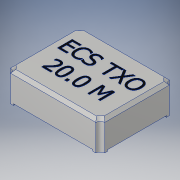
# Autodesk Inventor part: Crystal_TXO-3225
Saved by Autodesk Inventor 2018 (Build 220112000, 112)
## iProperties
Created: 2016-08-15
Part Number: Crystal_TXO-3225
Material: Aluminum 6061
Document SubType Name: Modeling
Designer: Bradley
Density: 2.7 g/cm^3
Appearance: Aluminum - Flat
Author: Bradley
Autodesk Inventor part; units mm, degrees
ref_plane "YZ Plane" through (0, 0, 0) normal (1, 0, 0) x (0, 1, 0)
ref_plane "XZ Plane" through (0, 0, 0) normal (0, 1, 0) x (-1, 0, 0)
ref_plane "XY Plane" through (0, 0, 0) normal (0, 0, 1) x (1, 0, 0)
sketch "Sketch1" plane through (0, 0, 0) normal (0, 1, 0) x (-1, 0, 0)
  line L0 (-1.6, 1.25) -> (1.6, 1.25)
  line L1 (1.6, 1.25) -> (1.6, -1.25)
  line L2 (1.6, -1.25) -> (-1.6, -1.25)
  line L3 (-1.6, -1.25) -> (-1.6, 1.25)
  line L4 (-1.6, 1.25) -> (1.6, -1.25) construction
  line L5 (1.6, 1.25) -> (-1.6, -1.25) construction
  arc A0 (1.6, -1.1) -> (1.45, -1.25) centre (1.6, -1.25) ccw
  arc A1 (-1.45, -1.25) -> (-1.6, -1.1) centre (-1.6, -1.25) ccw
  arc A2 (-1.6, 1.1) -> (-1.45, 1.25) centre (-1.6, 1.25) ccw
  arc A3 (1.45, 1.25) -> (1.6, 1.1) centre (1.6, 1.25) ccw
  point P0 (0, 0)
  dimension "d0" = 3.2
  dimension "d1" = 2.5
  dimension "d4" = 0.15
  constraints: 12 end point, 8 point on circle, 8 point on line, 4 centre point, 4 coincident, 3 equal radius, 2 midpoint, 2 parallel, 1 horizontal, 1 perpendicular
  measures "d0" distance of L1.end L2.end
  measures "d1" distance of L0.end L1.end
  measures "d4" radius of A0
extrude "Extrusion1" add sketch "Sketch1" along normal mid plane 0.95 contours L0 A3 L1 A0 L2 A1 L3 A2
chamfer "Chamfer1" distance 0.1 angle 45 8 edges at (0, 0.475, 1.25) (-1.4939, 0.475, 1.1439) (-1.6, 0.475, 0) (-1.4939, 0.475, -1.1439) (0, 0.475, -1.25) (1.4939, 0.475, -1.1439) (1.6, 0.475, 0) (1.4939, 0.475, 1.1439)
sketch "Sketch3" plane through (0, 0.475, 0) normal (0, 1, 0) x (1, 0, 0)
  line L0 (-1.3709, 1.15) -> (1.3709, 1.15) projected
  arc A0 (-1.5, 1.0209) -> (-1.3709, 1.15) centre (-1.6, 1.25) ccw projected
  line L1 (-1.5, -1.0209) -> (-1.5, 1.0209) projected
  arc A1 (-1.3709, -1.15) -> (-1.5, -1.0209) centre (-1.6, -1.25) ccw projected
  line L2 (1.3709, -1.15) -> (-1.3709, -1.15) projected
  arc A2 (1.5, -1.0209) -> (1.3709, -1.15) centre (1.6, -1.25) ccw projected
  line L3 (1.5, 1.0209) -> (1.5, -1.0209) projected
  arc A3 (1.3709, 1.15) -> (1.5, 1.0209) centre (1.6, 1.25) ccw projected
  line L4 (1.5, 1.0209) -> (1.5, -1.0209) construction
  line L5 (1.5, 0.1868) -> (-1.5, 0.1868) construction
  line L6 (-1.2911, 0.1868) -> (-1.2911, 0.6868)
  line L7 (-1.2911, 0.6868) -> (-0.9783, 0.6868)
  line L8 (-0.9783, 0.6868) -> (-0.9783, 0.6276)
  line L9 (-0.9783, 0.6276) -> (-1.2247, 0.6276)
  line L10 (-1.2247, 0.6276) -> (-1.2247, 0.4906)
  line L11 (-1.2247, 0.4906) -> (-0.9949, 0.4906)
  line L12 (-0.9949, 0.4906) -> (-0.9949, 0.4315)
  line L13 (-0.9949, 0.4315) -> (-1.2247, 0.4315)
  line L14 (-1.2247, 0.4315) -> (-1.2247, 0.2459)
  line L15 (-1.2247, 0.2459) -> (-0.9783, 0.2459)
  line L16 (-0.9783, 0.2459) -> (-0.9783, 0.1868)
  line L17 (-0.9783, 0.1868) -> (-1.2911, 0.1868)
  spline S0 degree 2 poles (-0.7101, 0.1778) (-0.7587, 0.1778) (-0.841, 0.2107) (-0.8709, 0.2435) knots 0 0 0 1 2 2 2
  spline S1 degree 2 poles (-0.8709, 0.2435) (-0.9009, 0.2759) (-0.9338, 0.3731) (-0.9338, 0.4364) knots 0 0 0 1 2 2 2
  spline S2 degree 2 poles (-0.9338, 0.4364) (-0.9338, 0.4992) (-0.9017, 0.5923) (-0.8714, 0.6268) knots 0 0 0 1 2 2 2
  spline S3 degree 2 poles (-0.8714, 0.6268) (-0.8414, 0.6604) (-0.7595, 0.6957) (-0.7089, 0.6957) knots 0 0 0 1 2 2 2
  spline S4 degree 2 poles (-0.7089, 0.6957) (-0.6838, 0.6957) (-0.6396, 0.6884) (-0.6209, 0.6827) knots 0 0 0 1 2 2 2
  spline S5 degree 2 poles (-0.6209, 0.6827) (-0.6047, 0.6774) (-0.5711, 0.6624) (-0.5545, 0.6535) knots 0 0 0 1 2 2 2
  line L18 (-0.5545, 0.6535) -> (-0.5545, 0.5733)
  line L19 (-0.5545, 0.5733) -> (-0.5598, 0.5733)
  spline S6 degree 2 poles (-0.5598, 0.5733) (-0.5687, 0.5814) (-0.5962, 0.6041) (-0.6161, 0.615) knots 0 0 0 1 2 2 2
  spline S7 degree 2 poles (-0.6161, 0.615) (-0.6351, 0.6256) (-0.6801, 0.6389) (-0.7093, 0.6389) knots 0 0 0 1 2 2 2
  spline S8 degree 2 poles (-0.7093, 0.6389) (-0.7413, 0.6389) (-0.7984, 0.6126) (-0.8199, 0.5875) knots 0 0 0 1 2 2 2
  spline S9 degree 2 poles (-0.8199, 0.5875) (-0.841, 0.562) (-0.8645, 0.4846) (-0.8645, 0.4364) knots 0 0 0 1 2 2 2
  spline S10 degree 2 poles (-0.8645, 0.4364) (-0.8645, 0.3849) (-0.8397, 0.3107) (-0.8183, 0.2852) knots 0 0 0 1 2 2 2
  spline S11 degree 2 poles (-0.8183, 0.2852) (-0.7972, 0.2605) (-0.7409, 0.2354) (-0.7093, 0.2354) knots 0 0 0 1 2 2 2
  spline S12 degree 2 poles (-0.7093, 0.2354) (-0.6805, 0.2354) (-0.6315, 0.2496) (-0.6124, 0.2601) knots 0 0 0 1 2 2 2
  spline S13 degree 2 poles (-0.6124, 0.2601) (-0.5942, 0.2706) (-0.5671, 0.2925) (-0.5594, 0.3002) knots 0 0 0 1 2 2 2
  line L20 (-0.5594, 0.3002) -> (-0.5545, 0.3002)
  line L21 (-0.5545, 0.3002) -> (-0.5545, 0.2208)
  spline S14 degree 2 poles (-0.5545, 0.2208) (-0.5711, 0.2131) (-0.6003, 0.1989) (-0.6209, 0.1924) knots 0 0 0 1 2 2 2
  spline S15 degree 2 poles (-0.6209, 0.1924) (-0.6428, 0.1851) (-0.6801, 0.1778) (-0.7101, 0.1778) knots 0 0 0 1 2 2 2
  spline S16 degree 2 poles (-0.3531, 0.1778) (-0.4074, 0.1778) (-0.4836, 0.2005) (-0.5172, 0.2167) knots 0 0 0 1 2 2 2
  line L22 (-0.5172, 0.2167) -> (-0.5172, 0.3002)
  line L23 (-0.5172, 0.3002) -> (-0.5124, 0.3002)
  spline S17 degree 2 poles (-0.5124, 0.3002) (-0.4795, 0.2694) (-0.3965, 0.2354) (-0.358, 0.2354) knots 0 0 0 1 2 2 2
  spline S18 degree 2 poles (-0.358, 0.2354) (-0.3029, 0.2354) (-0.2466, 0.2812) (-0.2466, 0.3188) knots 0 0 0 1 2 2 2
  spline S19 degree 2 poles (-0.2466, 0.3188) (-0.2466, 0.3488) (-0.2761, 0.3861) (-0.3081, 0.3954) knots 0 0 0 1 2 2 2
  spline S20 degree 2 poles (-0.3081, 0.3954) (-0.3312, 0.4019) (-0.3697, 0.4108) (-0.3985, 0.4181) knots 0 0 0 1 2 2 2
  spline S21 degree 2 poles (-0.3985, 0.4181) (-0.4244, 0.425) (-0.4654, 0.4457) (-0.4812, 0.4623) knots 0 0 0 1 2 2 2
  spline S22 degree 2 poles (-0.4812, 0.4623) (-0.4966, 0.4789) (-0.5136, 0.5235) (-0.5136, 0.5526) knots 0 0 0 1 2 2 2
  spline S23 degree 2 poles (-0.5136, 0.5526) (-0.5136, 0.6134) (-0.4188, 0.6957) (-0.3454, 0.6957) knots 0 0 0 1 2 2 2
  spline S24 degree 2 poles (-0.3454, 0.6957) (-0.3033, 0.6957) (-0.2287, 0.6791) (-0.1967, 0.6633) knots 0 0 0 1 2 2 2
  line L24 (-0.1967, 0.6633) -> (-0.1967, 0.5838)
  line L25 (-0.1967, 0.5838) -> (-0.2016, 0.5838)
  spline S25 degree 2 poles (-0.2016, 0.5838) (-0.2255, 0.6057) (-0.3, 0.6381) (-0.341, 0.6381) knots 0 0 0 1 2 2 2
  spline S26 degree 2 poles (-0.341, 0.6381) (-0.3872, 0.6381) (-0.4443, 0.5948) (-0.4443, 0.5595) knots 0 0 0 1 2 2 2
  spline S27 degree 2 poles (-0.4443, 0.5595) (-0.4443, 0.5279) (-0.4107, 0.4902) (-0.3791, 0.4817) knots 0 0 0 1 2 2 2
  spline S28 degree 2 poles (-0.3791, 0.4817) (-0.358, 0.4761) (-0.2968, 0.4615) (-0.2765, 0.4554) knots 0 0 0 1 2 2 2
  spline S29 degree 2 poles (-0.2765, 0.4554) (-0.2251, 0.4396) (-0.1773, 0.376) (-0.1773, 0.3294) knots 0 0 0 1 2 2 2
  spline S30 degree 2 poles (-0.1773, 0.3294) (-0.1773, 0.2998) (-0.2012, 0.2431) (-0.2226, 0.2232) knots 0 0 0 1 2 2 2
  spline S31 degree 2 poles (-0.2226, 0.2232) (-0.2466, 0.2013) (-0.3073, 0.1778) (-0.3531, 0.1778) knots 0 0 0 1 2 2 2
  line L26 (0.2218, 0.1868) -> (0.2218, 0.6276)
  line L27 (0.2218, 0.6276) -> (0.0541, 0.6276)
  line L28 (0.0541, 0.6276) -> (0.0541, 0.6868)
  line L29 (0.0541, 0.6868) -> (0.456, 0.6868)
  line L30 (0.456, 0.6868) -> (0.456, 0.6276)
  line L31 (0.456, 0.6276) -> (0.2883, 0.6276)
  line L32 (0.2883, 0.6276) -> (0.2883, 0.1868)
  line L33 (0.2883, 0.1868) -> (0.2218, 0.1868)
  line L34 (0.8527, 0.1868) -> (0.7765, 0.1868)
  line L35 (0.7765, 0.1868) -> (0.655, 0.3861)
  line L36 (0.655, 0.3861) -> (0.531, 0.1868)
  line L37 (0.531, 0.1868) -> (0.4593, 0.1868)
  line L38 (0.4593, 0.1868) -> (0.6185, 0.4372)
  line L39 (0.6185, 0.4372) -> (0.4641, 0.6868)
  line L40 (0.4641, 0.6868) -> (0.5403, 0.6868)
  line L41 (0.5403, 0.6868) -> (0.6594, 0.4911)
  line L42 (0.6594, 0.4911) -> (0.781, 0.6868)
  line L43 (0.781, 0.6868) -> (0.8527, 0.6868)
  line L44 (0.8527, 0.6868) -> (0.6963, 0.4404)
  line L45 (0.6963, 0.4404) -> (0.8527, 0.1868)
  spline S32 degree 2 poles (1.2599, 0.6296) (1.2883, 0.5964) (1.3199, 0.4992) (1.3199, 0.4368) knots 0 0 0 1 2 2 2
  spline S33 degree 2 poles (1.3199, 0.4368) (1.3199, 0.376) (1.2891, 0.2775) (1.2599, 0.2443) knots 0 0 0 1 2 2 2
  spline S34 degree 2 poles (1.2599, 0.2443) (1.2291, 0.2094) (1.1477, 0.1762) (1.0987, 0.1762) knots 0 0 0 1 2 2 2
  spline S35 degree 2 poles (1.0987, 0.1762) (1.048, 0.1762) (0.967, 0.2107) (0.9374, 0.2443) knots 0 0 0 1 2 2 2
  spline S36 degree 2 poles (0.9374, 0.2443) (0.9086, 0.2775) (0.8778, 0.3752) (0.8778, 0.4368) knots 0 0 0 1 2 2 2
  spline S37 degree 2 poles (0.8778, 0.4368) (0.8778, 0.4996) (0.909, 0.5952) (0.9378, 0.6296) knots 0 0 0 1 2 2 2
  spline S38 degree 2 poles (0.9378, 0.6296) (0.967, 0.6629) (1.0484, 0.6973) (1.0987, 0.6973) knots 0 0 0 1 2 2 2
  spline S39 degree 2 poles (1.0987, 0.6973) (1.1497, 0.6973) (1.2316, 0.6616) (1.2599, 0.6296) knots 0 0 0 1 2 2 2
  spline S40 degree 2 poles (1.2506, 0.4368) (1.2506, 0.4862) (1.2291, 0.5628) (1.2097, 0.5879) knots 0 0 0 1 2 2 2
  spline S41 degree 2 poles (1.2097, 0.5879) (1.1898, 0.6138) (1.1339, 0.6398) (1.0991, 0.6398) knots 0 0 0 1 2 2 2
  spline S42 degree 2 poles (1.0991, 0.6398) (1.063, 0.6398) (1.0087, 0.6146) (0.988, 0.5879) knots 0 0 0 1 2 2 2
  spline S43 degree 2 poles (0.988, 0.5879) (0.9682, 0.5624) (0.9471, 0.4854) (0.9471, 0.4368) knots 0 0 0 1 2 2 2
  spline S44 degree 2 poles (0.9471, 0.4368) (0.9471, 0.3383) (1.0298, 0.2338) (1.0991, 0.2338) knots 0 0 0 1 2 2 2
  spline S45 degree 2 poles (1.0991, 0.2338) (1.1684, 0.2338) (1.2506, 0.3383) (1.2506, 0.4368) knots 0 0 0 1 2 2 2
  line L46 (-0.6945, -0.6389) -> (-1.0028, -0.6389)
  line L47 (-1.0028, -0.6389) -> (-1.0028, -0.568)
  spline S46 degree 2 poles (-1.0028, -0.568) (-0.9696, -0.5368) (-0.9105, -0.4789) (-0.8821, -0.4477) knots 0 0 0 1 2 2 2
  spline S47 degree 2 poles (-0.8821, -0.4477) (-0.825, -0.3849) (-0.7832, -0.3095) (-0.7832, -0.2694) knots 0 0 0 1 2 2 2
  spline S48 degree 2 poles (-0.7832, -0.2694) (-0.7832, -0.2483) (-0.7962, -0.2167) (-0.8079, -0.2066) knots 0 0 0 1 2 2 2
  spline S49 degree 2 poles (-0.8079, -0.2066) (-0.8197, -0.1965) (-0.8505, -0.1863) (-0.8691, -0.1863) knots 0 0 0 1 2 2 2
  spline S50 degree 2 poles (-0.8691, -0.1863) (-0.887, -0.1863) (-0.9234, -0.1952) (-0.94, -0.2021) knots 0 0 0 1 2 2 2
  spline S51 degree 2 poles (-0.94, -0.2021) (-0.9542, -0.2078) (-0.9806, -0.224) (-0.9887, -0.2297) knots 0 0 0 1 2 2 2
  line L48 (-0.9887, -0.2297) -> (-0.9923, -0.2297)
  line L49 (-0.9923, -0.2297) -> (-0.9923, -0.1584)
  spline S52 degree 2 poles (-0.9923, -0.1584) (-0.9716, -0.1482) (-0.8975, -0.1284) (-0.8643, -0.1284) knots 0 0 0 1 2 2 2
  spline S53 degree 2 poles (-0.8643, -0.1284) (-0.7942, -0.1284) (-0.7152, -0.2025) (-0.7152, -0.2657) knots 0 0 0 1 2 2 2
  spline S54 degree 2 poles (-0.7152, -0.2657) (-0.7152, -0.2953) (-0.7289, -0.3448) (-0.7411, -0.3658) knots 0 0 0 1 2 2 2
  spline S55 degree 2 poles (-0.7411, -0.3658) (-0.7532, -0.3877) (-0.7885, -0.4307) (-0.8079, -0.4513) knots 0 0 0 1 2 2 2
  spline S56 degree 2 poles (-0.8079, -0.4513) (-0.8395, -0.4858) (-0.9169, -0.5595) (-0.94, -0.581) knots 0 0 0 1 2 2 2
  line L50 (-0.94, -0.581) -> (-0.6945, -0.581)
  line L51 (-0.6945, -0.581) -> (-0.6945, -0.6389)
  spline S57 degree 2 poles (-0.3165, -0.3889) (-0.3165, -0.5234) (-0.3947, -0.6495) (-0.4761, -0.6495) knots 0 0 0 1 2 2 2
  spline S58 degree 2 poles (-0.4761, -0.6495) (-0.5588, -0.6495) (-0.6361, -0.521) (-0.6361, -0.3893) knots 0 0 0 1 2 2 2
  spline S59 degree 2 poles (-0.6361, -0.3893) (-0.6361, -0.254) (-0.5579, -0.1288) (-0.4761, -0.1288) knots 0 0 0 1 2 2 2
  spline S60 degree 2 poles (-0.4761, -0.1288) (-0.3938, -0.1288) (-0.3165, -0.2585) (-0.3165, -0.3889) knots 0 0 0 1 2 2 2
  spline S61 degree 2 poles (-0.4024, -0.5413) (-0.3926, -0.5166) (-0.3845, -0.4404) (-0.3845, -0.3889) knots 0 0 0 1 2 2 2
  spline S62 degree 2 poles (-0.3845, -0.3889) (-0.3845, -0.3375) (-0.3926, -0.2617) (-0.4028, -0.2362) knots 0 0 0 1 2 2 2
  spline S63 degree 2 poles (-0.4028, -0.2362) (-0.4129, -0.2106) (-0.4481, -0.1843) (-0.4761, -0.1843) knots 0 0 0 1 2 2 2
  spline S64 degree 2 poles (-0.4761, -0.1843) (-0.5041, -0.1843) (-0.5401, -0.2106) (-0.5506, -0.237) knots 0 0 0 1 2 2 2
  spline S65 degree 2 poles (-0.5506, -0.237) (-0.5608, -0.2625) (-0.5681, -0.3403) (-0.5681, -0.3893) knots 0 0 0 1 2 2 2
  spline S66 degree 2 poles (-0.5681, -0.3893) (-0.5681, -0.442) (-0.5616, -0.5125) (-0.5511, -0.5401) knots 0 0 0 1 2 2 2
  spline S67 degree 2 poles (-0.5511, -0.5401) (-0.5413, -0.566) (-0.5053, -0.5939) (-0.4761, -0.5939) knots 0 0 0 1 2 2 2
  spline S68 degree 2 poles (-0.4761, -0.5939) (-0.4485, -0.5939) (-0.4125, -0.5676) (-0.4024, -0.5413) knots 0 0 0 1 2 2 2
  line L52 (-0.1451, -0.6389) -> (-0.2253, -0.6389)
  line L53 (-0.2253, -0.6389) -> (-0.2253, -0.5433)
  line L54 (-0.2253, -0.5433) -> (-0.1451, -0.5433)
  line L55 (-0.1451, -0.5433) -> (-0.1451, -0.6389)
  spline S69 degree 2 poles (0.267, -0.3889) (0.267, -0.5234) (0.1888, -0.6495) (0.1074, -0.6495) knots 0 0 0 1 2 2 2
  spline S70 degree 2 poles (0.1074, -0.6495) (0.0247, -0.6495) (-0.0527, -0.521) (-0.0527, -0.3893) knots 0 0 0 1 2 2 2
  spline S71 degree 2 poles (-0.0527, -0.3893) (-0.0527, -0.254) (0.0255, -0.1288) (0.1074, -0.1288) knots 0 0 0 1 2 2 2
  spline S72 degree 2 poles (0.1074, -0.1288) (0.1896, -0.1288) (0.267, -0.2585) (0.267, -0.3889) knots 0 0 0 1 2 2 2
  spline S73 degree 2 poles (0.1811, -0.5413) (0.1908, -0.5166) (0.1989, -0.4404) (0.1989, -0.3889) knots 0 0 0 1 2 2 2
  spline S74 degree 2 poles (0.1989, -0.3889) (0.1989, -0.3375) (0.1908, -0.2617) (0.1807, -0.2362) knots 0 0 0 1 2 2 2
  spline S75 degree 2 poles (0.1807, -0.2362) (0.1706, -0.2106) (0.1353, -0.1843) (0.1074, -0.1843) knots 0 0 0 1 2 2 2
  spline S76 degree 2 poles (0.1074, -0.1843) (0.0794, -0.1843) (0.0434, -0.2106) (0.0328, -0.237) knots 0 0 0 1 2 2 2
  spline S77 degree 2 poles (0.0328, -0.237) (0.0227, -0.2625) (0.0154, -0.3403) (0.0154, -0.3893) knots 0 0 0 1 2 2 2
  spline S78 degree 2 poles (0.0154, -0.3893) (0.0154, -0.442) (0.0219, -0.5125) (0.0324, -0.5401) knots 0 0 0 1 2 2 2
  spline S79 degree 2 poles (0.0324, -0.5401) (0.0421, -0.566) (0.0782, -0.5939) (0.1074, -0.5939) knots 0 0 0 1 2 2 2
  spline S80 degree 2 poles (0.1074, -0.5939) (0.1349, -0.5939) (0.171, -0.5676) (0.1811, -0.5413) knots 0 0 0 1 2 2 2
  line L56 (0.9887, -0.6389) -> (0.9222, -0.6389)
  line L57 (0.9222, -0.6389) -> (0.9222, -0.2082)
  line L58 (0.9222, -0.2082) -> (0.7917, -0.5012)
  line L59 (0.7917, -0.5012) -> (0.7512, -0.5012)
  line L60 (0.7512, -0.5012) -> (0.622, -0.2082)
  line L61 (0.622, -0.2082) -> (0.622, -0.6389)
  line L62 (0.622, -0.6389) -> (0.56, -0.6389)
  line L63 (0.56, -0.6389) -> (0.56, -0.1389)
  line L64 (0.56, -0.1389) -> (0.6507, -0.1389)
  line L65 (0.6507, -0.1389) -> (0.7755, -0.4173)
  line L66 (0.7755, -0.4173) -> (0.8963, -0.1389)
  line L67 (0.8963, -0.1389) -> (0.9887, -0.1389)
  line L68 (0.9887, -0.1389) -> (0.9887, -0.6389)
  point P0 (0, 0)
  constraints: 2 end point, 2 point on line, 1 horizontal, 1 perpendicular
extrude "Extrusion3" add sketch "Sketch3" along normal blind 0.01 contours L6 L7 L8 L9 L10 L11 L12 L13 L14 L15 L16 L17 | S0 S1 S2 S3 S4 S5 L18 L19 S6 S7 S8 S9 S10 S11 S12 S13 L20 L21 S14 S15 | S16 L22 L23 S17 S18 S19 S20 S21 S22 S23 S24 L24 L25 S25 S26 S27 S28 S29 S30 S31 | L26 L27 L28 L29 L30 L31 L32 L33 | L34 L35 L36 L37 L38 L39 L40 L41 L42 L43 L44 L45 | S32 S33 S34 S35 S36 S37 S38 S39 | L46 L47 S46 S47 S48 S49 S50 S51 L48 L49 S52 S53 S54 S55 S56 L50 L51 | S57 S58 S59 S60 | L52 L53 L54 L55 | S69 S70 S71 S72 | L56 L57 L58 L59 L60 L61 L62 L63 L64 L65 L66 L67 L68
sketch "Sketch4" plane through (0, -0.475, 0) normal (0, -1, 0) x (1, 0, 0)
  line L0 (-1.6, 1.1) -> (-1.6, -1.1) projected
  arc A0 (-1.45, -1.25) -> (-1.6, -1.1) centre (-1.6, -1.25) ccw projected
  line L1 (-1.45, -1.25) -> (1.45, -1.25) projected
  arc A1 (1.6, -1.1) -> (1.45, -1.25) centre (1.6, -1.25) ccw projected
  line L2 (1.6, -1.1) -> (1.6, 1.1) projected
  arc A2 (1.45, 1.25) -> (1.6, 1.1) centre (1.6, 1.25) ccw projected
  line L3 (1.45, 1.25) -> (-1.45, 1.25) projected
  arc A3 (-1.6, 1.1) -> (-1.45, 1.25) centre (-1.6, 1.25) ccw projected
  line L4 (1.35, 1.25) -> (1.35, 1.19)
  line L5 (1.35, 1.19) -> (0.94, 1.19)
  line L6 (0.94, 1.19) -> (0.94, 0.35)
  line L7 (0.94, 0.35) -> (1.54, 0.35)
  line L8 (1.54, 0.35) -> (1.54, 1)
  line L9 (1.54, 1) -> (1.6, 1)
  line L10 (-1.6, -1.1) -> (-1.6, 1.1) projected
  line L11 (-1.6, 1) -> (-1.54, 1)
  line L12 (-1.54, 1) -> (-1.54, 0.35)
  line L13 (-1.54, 0.35) -> (-0.94, 0.35)
  line L14 (-0.94, 0.35) -> (-0.94, 1.19)
  line L15 (-0.94, 1.19) -> (-1.35, 1.19)
  line L16 (-1.35, 1.19) -> (-1.35, 1.25)
  line L17 (1.45, -1.25) -> (-1.45, -1.25) projected
  line L18 (-1.35, -1.25) -> (-1.35, -1.19)
  line L19 (-1.35, -1.19) -> (-0.94, -1.19)
  line L20 (-0.94, -1.19) -> (-0.94, -0.35)
  line L21 (-0.94, -0.35) -> (-1.54, -0.35)
  line L22 (-1.54, -0.35) -> (-1.54, -1)
  line L23 (-1.54, -1) -> (-1.6, -1)
  line L24 (1.6, -1) -> (1.54, -1)
  line L25 (1.54, -1) -> (1.54, -0.35)
  line L26 (1.54, -0.35) -> (0.94, -0.35)
  line L27 (0.94, -0.35) -> (0.94, -1.19)
  line L28 (0.94, -1.19) -> (1.35, -1.19)
  line L29 (1.35, -1.19) -> (1.35, -1.25)
  point P0 (0, 0)
  dimension "d20" = 0.84
  dimension "d21" = 0.6
  dimension "d22" = 1.88
  dimension "d23" = 0.25
  dimension "d24" = 0.25
  constraints: 48 end point, 20 point on line, 15 perpendicular, 7 equal length, 6 collinear, 1 horizontal, 1 parallel, 1 vertical
  measures "d20" distance of L5.end L6.end
  measures "d21" distance of L6.end L7.end
  measures "d22" distance between parallel lines of L14 L6
  measures "d23" distance between parallel lines of L4 L2
  measures "d24" distance between parallel lines of L9 L3
extrude "Extrusion5" add sketch "Sketch4" along normal blind 0.05 contours A3 L3 L16 L15 L14 L13 L12 L11 L0 | L23 L22 L21 L20 L19 L18 L1 A0 L0 | L3 A2 L2 L9 L8 L7 L6 L5 L4 | L29 L28 L27 L26 L25 L24 L2 A1 L1
equation "\"d24\" = d23"
body "Solid1"
